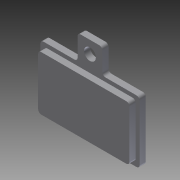
# Autodesk Inventor part: lid
Saved by Autodesk Inventor 2011 (Build 150239000, 239)
## iProperties
Created: 2011-02-17
Part Number: lid
Document SubType Name: Modeling
Designer: labuser
Density: 1 g/cm^3
Author: labuser
Autodesk Inventor part; units mm, degrees
ref_plane "YZ Plane" through (0, 0, 0) normal (1, 0, 0) x (0, 1, 0)
ref_plane "XZ Plane" through (0, 0, 0) normal (0, 1, 0) x (-1, 0, 0)
ref_plane "XY Plane" through (0, 0, 0) normal (0, 0, 1) x (1, 0, 0)
sketch "Sketch1" plane through (0, 0, 0) normal (0, 0, 1) x (1, 0, 0)
  line L0 (0, 0) -> (16, 0)
  line L1 (16, 0) -> (16, 10)
  line L2 (16, 10) -> (0, 10)
  line L3 (0, 10) -> (0, 0)
  dimension "d0" = 16
  dimension "d1" = 10
  constraints: 8 end point, 2 parallel, 1 horizontal, 1 perpendicular
  measures "d0" distance of L2.end L1.end
  measures "d1" distance of L1.end L0.end
extrude "Extrusion1" add sketch "Sketch1" along normal blind 2
sketch "Sketch2" plane through (0, 0, 2) normal (0, 0, 1) x (1, 0, 0)
  line L0 (0, 0) -> (0, 10) projected
  line L1 (16, 0) -> (0, 0) projected
  line L2 (16, 10) -> (16, 0) projected
  line L3 (0, 10) -> (16, 10) projected
  line L4 (0.635, 9.365) -> (0.635, 0.635)
  line L5 (0.635, 0.635) -> (15.365, 0.635)
  line L6 (15.365, 0.635) -> (15.365, 9.365)
  line L7 (15.365, 9.365) -> (0.635, 9.365)
  dimension "d4" = 0.635
  constraints: 8 end point, 3 other
  measures "d4" distance between parallel lines of L0 L4
extrude "Extrusion2" cut sketch "Sketch2" against normal blind 1
sketch "Sketch3" plane through (0, 10, 0) normal (0, 1, 0) x (1, 0, 0)
  line L0 (0, -1) -> (16, -1) projected
  line L1 (16, 0) -> (0, 0) projected
  line L2 (0, 0) -> (0, -1) projected
  line L3 (6, 0) -> (10, 0)
  line L4 (10, 0) -> (10, -1)
  line L5 (10, -1) -> (6, -1)
  line L6 (6, -1) -> (6, 0)
  dimension "d7" = 4
  dimension "d8" = 6
  constraints: 8 end point, 2 parallel, 2 point on line, 1 horizontal, 1 perpendicular
  measures "d7" distance of L4.end L5.end
  measures "d8" distance between parallel lines of L6 L2
extrude "Extrusion3" add sketch "Sketch3" along normal blind 4 contours L6 L1 L4 L0
sketch "Sketch4" plane through (0, 0, 1) normal (0, 0, 1) x (1, 0, 0)
  point P0 (8, 12)
hole "Hole1" at (8, 12, 1) direction (0, 0, -1) diameter 1.905 end through all
fillet "Fillet1" radius 0.5 12 edges at (0.635, 0.635, 1.5) (0, 0, 0.5) (0.635, 9.365, 1.5) (0, 10, 0.5) (15.365, 0.635, 1.5) (16, 0, 0.5) (15.365, 9.365, 1.5) (16, 10, 0.5) (10, 10, 0.5) (6, 10, 0.5) (6, 14, 0.5) (10, 14, 0.5)
body "Solid1"
